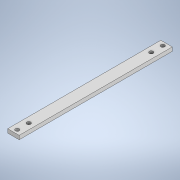
# Autodesk Inventor part: camera_arm
Saved by Autodesk Inventor 2020 (Build 240168000, 168)
## iProperties
Created: 2020-02-14
Part Number: camera_arm
Material: Generic
Document SubType Name: Modeling
Designer: mdjb501
Density: 1 g/cm^3
Appearance: Default
Author: mdjb501
Autodesk Inventor part; units mm, degrees
ref_plane "YZ Plane" through (0, 0, 0) normal (1, 0, 0) x (0, 1, 0)
ref_plane "XZ Plane" through (0, 0, 0) normal (0, 1, 0) x (-1, 0, 0)
ref_plane "XY Plane" through (0, 0, 0) normal (0, 0, 1) x (1, 0, 0)
sketch "Sketch1" plane through (0, 0, 0) normal (0, 1, 0) x (-1, 0, 0)
  line L0 (-3, 40) -> (3, 40)
  line L1 (3, 40) -> (3, -40)
  line L2 (3, -40) -> (-3, -40)
  line L3 (-3, -40) -> (-3, 40)
  circle A0 centre (0, 38) radius 1
  circle A1 centre (0, 32) radius 1
  circle A2 centre (0, -32) radius 1
  circle A3 centre (0, -38) radius 1
  point P0 (0, 0)
  constraints: 8 end point, 4 centre point, 2 parallel, 1 horizontal, 1 perpendicular
extrude "Extrusion1" add sketch "Sketch1" along normal blind 2
body "Solid1"
